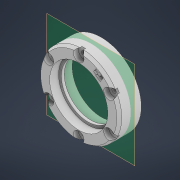
# Autodesk Inventor part: Ring Cover Top
Saved by Autodesk Inventor 2021 (Build 250183000, 183)
## iProperties
Created: 2025-03-19
Part Number: Ring Cover Top
Material: Generic
Document SubType Name: Modeling
Designer: rocke
Density: 0.528258 g/cm^3
Appearance: Default
Mass: 26.1 g
Surface Area: 167.965 cm^2
Volume: 49.4077 cm^3
Author: rocke
Autodesk Inventor part; units mm, degrees
ref_plane "YZ Plane" through (0, 0, 0) normal (1, 0, 0) x (0, 1, 0)
ref_plane "XZ Plane" through (0, 0, 0) normal (0, 1, 0) x (-1, 0, 0)
ref_plane "XY Plane" through (0, 0, 0) normal (0, 0, 1) x (1, 0, 0)
sketch "Sketch1" plane through (0, 0, 0) normal (0, 0, 1) x (1, 0, 0)
  circle A0 centre (0, 0) radius 40
  dimension "d0" = 80
  constraints: 1 centre point, 1 coincident
  measures "d0" diameter of A0
extrude "Extrusion1" add sketch "Sketch1" along normal blind 22.5
sketch "Sketch2" plane through (0, 0, 22.5) normal (0, 0, 1) x (1, 0, 0)
  point P0 (0, 0)
  point P1 (0, 35)
  dimension "d3" = 35
  measures "d3" distance of point (0, 0) point (0, 35)
hole "Hole1" at (0, 35, 22.5) direction (0, 0, -1) diameter 4.3 end through all counterbore diameter 10.59 counterbore depth 5 clearance for "Hex Head Machine Screw" size "M4" standard "Ansi Metric M Profile"
chamfer "Chamfer1" distance 2 distance2 3 2 edges at (-27.6179, -28.9353, 22.5) (28.9353, 27.6179, 22.5) measured on face at (-2.7418, -16.4668, 22.5)
pattern_circular "Circular Pattern1" count 6 over 360 about axis through (0, 0, 0) along (0, 0, 1) of "Hole1"
sketch "Sketch3" plane through (0, 0, 0) normal (0, 0, -1) x (-1, 0, 0)
  circle A0 centre (0, 0) radius 29.1
  dimension "d17" = 58.2
  constraints: 1 centre point, 1 coincident
  measures "d17" diameter of A0
extrude "Extrusion2" cut sketch "Sketch3" against normal through all
ref_plane "Work Plane1" through (0, 0, 10.5) normal (0, 0, -1) x (-1, 0, 0)
sketch "Sketch4" plane through (0, 0, 10.5) normal (0, 0, -1) x (-1, 0, 0)
  circle A0 centre (0, 0) radius 29.5
  circle A1 centre (0, 0) radius 26.5
  dimension "d21" = 53
  dimension "d22" = 59
  constraints: 2 centre point, 2 coincident
  measures "d21" diameter of A1
  measures "d22" diameter of A0
extrude "Extrusion3" add sketch "Sketch4" against normal blind 3
sketch "Sketch5" plane through (0, 0, 22.5) normal (0, 0, 1) x (1, 0, 0)
  arc A0 (33.6722, 21.5913) -> (1.8625, 39.9566) centre (0, 0) ccw projected
  line L0 (0, 0) -> (40, 0) construction
  line L1 (21.4926, 23.7527) -> (24.6091, 28.2845)
  line L2 (24.6091, 28.2845) -> (17.6054, 33.101)
  line L3 (17.6054, 33.101) -> (14.4889, 28.5691)
  line L4 (14.4889, 28.5691) -> (21.4926, 23.7527)
  line L5 (21.4926, 23.7527) -> (17.6054, 33.101) construction
  line L6 (24.6091, 28.2845) -> (14.4889, 28.5691) construction
  line L7 (17.002, 26.8409) -> (20.1185, 31.3727)
  line L8 (22.1372, 29.9845) -> (19.0207, 25.4526)
  line L9 (14.8714, 29.1253) -> (17.223, 32.5448)
  line L10 (17.223, 32.5448) -> (19.736, 30.8165)
  line L11 (19.736, 30.8165) -> (17.3845, 27.3971)
  line L12 (17.3845, 27.3971) -> (14.8714, 29.1253)
  line L13 (19.549, 28.4268) -> (16.0472, 30.8351)
  line L14 (17.3845, 27.3971) -> (17.223, 32.5448)
  line L15 (14.8714, 29.1253) -> (19.736, 30.8165)
  line L16 (0, 0) -> (17.3037, 29.9709)
  line L17 (0, 0) -> (19.549, 28.4268)
  dimension "d26" = 8.5
  dimension "d27" = 5.5
  dimension "d29" = 34.5
  dimension "d30" = 3.05
  dimension "d36" = 3
  dimension "d41" = 4.15
  dimension "d42" = 60
  constraints: 36 end point, 6 point on line, 5 parallel, 5 perpendicular, 4 midpoint, 1 collinear, 1 horizontal, 1 other
  measures "d26" distance between parallel lines of L1 L3
  measures "d27" distance between parallel lines of L4 L2
  measures "d29" distance of L16.start L13.start
  measures "d30" distance between parallel lines of L3 L7
  measures "d36" distance between parallel lines of L1 L8
  measures "d41" distance between parallel lines of L12 L10
  measures "d42" angle of L0 L16
extrude "Extrusion4" cut sketch "Sketch5" against normal blind 1.75 contours L4 L17 L13 L7 L2 L8 | L4 L7 L13 L17 | L15 L14 L10 | L7 L13 L15 | L14 L13 L7 | L12 L16 L14 | L14 L13 L3 | L15 L3 L13 | L16 L12 L15
extrude "Extrusion7" cut sketch "Sketch5" against normal through all contours L4 L8 L2 L1
body "Solid1"
